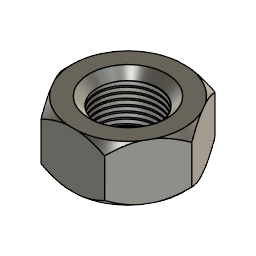
Hex_Nut (Autodesk Fusion 360 design; units mm, degrees)
Autodesk Fusion 360 part; units mm, degrees
note: some values were not read from the file. Chosen so that the rebuilt part matches the saved one: which face or edge a step refers to; where a thread starts.
sketch "Hex Polygon" plane through (0, 0, 0) normal (0, 0, 1) x (1, 0, 0)
  line L0 (5.7735, 10) -> (-5.7735, 10)
  line L1 (-5.7735, 10) -> (-11.547, 0)
  line L2 (-11.547, 0) -> (-5.7735, -10)
  line L3 (-5.7735, -10) -> (5.7735, -10)
  line L4 (5.7735, -10) -> (11.547, 0)
  line L5 (11.547, 0) -> (5.7735, 10)
  dimension "d1" = 10
  constraint horizontal L0
  measures "d1" distance of origin L5
extrude "Extrude1" add sketch "Hex Polygon" along normal blind 10
sketch "Chamfer Sketch" plane through (0, 0, 0) normal (0, 1, 0) x (1, 0, 0)
  line L0 (11.547, -10) -> (10.047, -10)
  line L1 (10.047, -10) -> (11.547, -8.5)
  line L2 (11.547, -8.5) -> (11.547, -10)
  point P0 (11.547, -10)
  dimension "d4" = 1.5
  constraint coincident P0 L0.start
  constraint horizontal L0
  constraint perpendicular L0 L2
  constraint equal L0 L2
  measures "d4" distance of L1.end P0
revolve "Revolve1" cut sketch "Chamfer Sketch" angle 360 about axis through (0, 0, 1.75) along (0, 0, 1)
hole "Hole1" at (0, 0, 10) direction (0, 0, -1) diameter 11.035 end through all countersink diameter 14 countersink angle 90
thread "Thread1" "GB Metric profile 12.0 M12x1 M12x1 6H" major diameter 12.152 minor diameter 11.035 pitch 1 angle 60 modelled right hand crest width 0.2719 on face at (0.5494, -5.4901, 2.8392) crest through (0, -5.5175, 9.0175)
ref_plane "WorkPlane1" through (0, 0, 5) normal (0, 0, 1) x (1, 0, 0)
mirror "Mirror1" about plane through (0, 0, 5) normal (0, 0, 1) of "Revolve1", "Hole1"
named bodies: "Hex Body"
